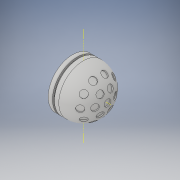
# Autodesk Inventor part: Pata - Pie
Saved by Autodesk Inventor 2019 (Build 230136000, 136)
## iProperties
Created: 2020-03-05
Part Number: Pata - Pie
Material: Genérico
Document SubType Name: Modeling
Designer: eddysanoli
Density: 1 g/cm^3
Appearance: Valor por defecto
Author: eddysanoli
Autodesk Inventor part; units mm, degrees
ref_plane "YZ Plane" through (0, 0, 0) normal (1, 0, 0) x (0, 1, 0)
ref_plane "XZ Plane" through (0, 0, 0) normal (0, 1, 0) x (-1, 0, 0)
ref_plane "XY Plane" through (0, 0, 0) normal (0, 0, 1) x (1, 0, 0)
sketch "Boceto1" plane through (0, 0, 0) normal (0, 1, 0) x (-1, 0, 0)
  line L0 (18.3875, 12.2875) -> (26.3875, 12.2875)
  line L1 (26.3875, -12.2875) -> (18.3875, -12.2875) construction
  line L2 (26.3875, 18.3875) -> (26.3875, 14.3875)
  line L3 (26.3875, 14.3875) -> (18.3875, 14.3875)
  line L4 (18.3875, 14.3875) -> (18.3875, 12.2875)
  line L5 (18.3875, -12.2875) -> (18.3875, -14.3875) construction
  line L6 (18.3875, -14.3875) -> (26.3875, -14.3875) construction
  line L7 (26.3875, -14.3875) -> (26.3875, -18.3875) construction
  line L8 (18.3875, 18.3875) -> (21.6375, 18.3875)
  line L9 (21.6375, 18.3875) -> (21.6375, 16.8875)
  line L10 (21.6375, 16.8875) -> (23.1375, 16.8875)
  line L11 (23.1375, 16.8875) -> (23.1375, 18.3875)
  line L12 (23.1375, 18.3875) -> (26.3875, 18.3875)
  line L13 (18.3875, -18.3875) -> (21.6375, -18.3875) construction
  line L14 (21.6375, -18.3875) -> (21.6375, -16.8875) construction
  line L15 (21.6375, -16.8875) -> (23.1375, -16.8875) construction
  line L16 (23.1375, -16.8875) -> (23.1375, -18.3875) construction
  line L17 (23.1375, -18.3875) -> (26.3875, -18.3875) construction
  line L18 (0, 0) -> (26.3875, 0)
  line L19 (26.3875, 12.2875) -> (26.3875, 0)
  line L20 (26.3875, 0) -> (26.3875, -12.2875) construction
  arc A0 (18.3875, 18.3875) -> (0, 0) centre (18.3875, 0) ccw
  arc A1 (0, 0) -> (18.3875, -18.3875) centre (18.3875, 0) ccw construction
  point P0 (26.3875, 16.3875)
  point P1 (26.3875, -16.3875)
  dimension "d0" = 24.575
  dimension "d3" = 2.1
  dimension "d4" = 4
  dimension "d5" = 8
  dimension "d6" = 1.5
  dimension "d8" = 3.25
  dimension "alto_esfera" = 18.3875
  constraints: 42 end point, 14 perpendicular, 8 equal length, 6 vertical alignment, 4 point on circle, 3 horizontal, 3 tangent, 2 centre point, 2 coincident, 2 midpoint, 2 point on line, 1 concentric, 1 vertical, 1 other
  measures "d0" distance of L0.end L1.start
  measures "d3" distance of L3.end L0.start
  measures "d4" distance of L2.start L2.end
  measures "d5" distance of L1.start L1.end
  measures "d6" distance of L8.end L9.end
  measures "d8" distance from line of L9 L8.start
  measures "alto_esfera" distance of point (0, 0) A0.centre
revolve "Revolución1" add sketch "Boceto1" angle 360 about axis through (0, 0, 0) along (-1, 0, 0)
ref_plane "Plano de trabajo1" through (0, 0, 0) normal (-1, 0, 0) x (0, -1, 0)
sketch "Boceto2" plane through (0, 0, 0) normal (-1, 0, 0) x (0, -1, 0)
  circle A0 centre (0, 0) radius 2.5
  dimension "d10" = 5
  constraints: 1 centre point, 1 coincident
  measures "d10" diameter of A0
extrude "Extrusión1" cut sketch "Boceto2" along normal blind 1
ref_plane "Plano de trabajo2" through (-18.3875, 0, 0) normal (-1, 0, 0) x (0, -1, 0)
sketch "Boceto3" plane through (-18.3875, 0, 0) normal (-1, 0, 0) x (0, -1, 0)
  line L0 (-32.5738, 0) -> (28.8087, 0) construction
  point P0 (0, 0)
  constraints: 2 end point, 1 horizontal
pattern_circular "Patrón circular1" count 2 over 25 about axis through (-18.3875, 32.5738, 0) along (0, -1, 0) of "Extrusión1"
pattern_circular "Patrón circular2" count 6 over 360 about axis through (-0.1707, 0, 0) along (-1, 0, 0) of "Extrusión1", "Patrón circular1"
pattern_circular "Patrón circular3" count 2 over 50 about axis through (-18.3875, 32.5738, 0) along (0, -1, 0) of "Extrusión1"
pattern_circular "Patrón circular4" count 10 over 360 about axis through (-0.1707, 0, 0) along (-1, 0, 0) of "Extrusión1", "Patrón circular3"
equation "\"d0\" = diametro_agujero_brazo"
equation "\"d3\" = 1.05 * grosor_pared_agujero_brazo"
equation "\"d5\" = profundidad_agujero_brazo"
equation "\"d8\" = -0.5 * d6 + 0.5 * d5"
equation "\"d14\" = alto_esfera"
equation "\"diametro_agujero_brazo\" = 24.575"
equation "\"grosor_pared_agujero_brazo\" = 2"
equation "\"profundidad_agujero_brazo\" = 8"
